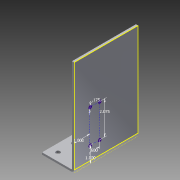
# Autodesk Inventor part: Pneumatic Mount Bracket
Saved by Autodesk Inventor 2013 (Build 170138000, 138)
## iProperties
Created: 2013-02-09
Part Number: Pneumatic Mount Bracket
Material: Aluminum 6061
Document SubType Name: Sheet Metal
Designer: Moses
Mass: 172.904 g
Surface Area: 422.955 cm^2
Volume: 63.8022 cm^3
Density: 2.71 g/cm^3
Sheet Metal Rule: Default
Author: Moses
Autodesk Inventor part; units mm, degrees
ref_plane "YZ Plane" through (0, 0, 0) normal (1, 0, 0) x (0, 1, 0)
ref_plane "XZ Plane" through (0, 0, 0) normal (0, 1, 0) x (-1, 0, 0)
ref_plane "XY Plane" through (0, 0, 0) normal (0, 0, 1) x (1, 0, 0)
sketch "Sketch1" plane through (0, 0, 0) normal (0, 1, 0) x (-1, 0, 0)
  line L0 (0, 0) -> (25.4, 0)
  line L1 (25.4, 0) -> (25.4, 101.6)
  line L2 (25.4, 101.6) -> (0, 101.6)
  line L3 (0, 101.6) -> (0, 0)
  line L4 (12.7, 101.6) -> (12.7, 0) construction
  circle A0 centre (12.7, 12.7) radius 3.302
  circle A1 centre (12.7, 63.5) radius 3.302
  circle A2 centre (12.7, 88.9) radius 3.302
  line L5 (0, 0) -> (-25.4, 0)
  line L6 (-25.4, 0) -> (-25.4, 101.6)
  line L7 (-25.4, 101.6) -> (0, 101.6)
  dimension "d0" = 101.6
  dimension "d2" = 25.4
  dimension "d3" = 6.604
  dimension "d4" = 25.4
  dimension "d5" = 50.8
  dimension "d6" = 12.7
  dimension "d8" = 25.4
  measures "d0" distance of L0.end L1.end
  measures "d2" distance of L0.start L0.end
  measures "d3" diameter of A2
  measures "d4" distance of A1.centre A2.centre
  measures "d5" distance of A0.centre A1.centre
  measures "d6" distance of L4.end A0.centre
  measures "d8" distance of L0.start L5.end
extrude "Plate1" add sketch "Sketch1" along normal blind 3.175
sketch "Sketch2" plane through (22.225, 0, 0) normal (1, 0, 0) x (0, 1, 0)
  line L0 (0, 101.6) -> (0, 0)
  line L1 (0, 0) -> (152.4, 0)
  line L2 (152.4, 0) -> (152.4, 101.6)
  line L3 (152.4, 101.6) -> (0, 101.6)
  constraints: 6 end point, 1 horizontal, 1 perpendicular, 1 vertical
edge flange "Flange1" height 152.4 angle 90 thickness 3.175 bend radius 1.27 thickness toward (1, 0, 0) relief tear relief width 3.175 relief depth 1.5875 edges at (25.4, 3.175, 50.8) wall of the first edge with corners at (22.225, 0, 101.6) (22.225, 0, 0) (22.225, 152.4, 0) (22.225, 152.4, 101.6)
bend "Bend1"
corner "Corner1"
sketch "Sketch3" plane through (25.4, 152.4, 101.6) normal (1, 0, 0) x (0, 0, -1)
  line L0 (0, -147.955) -> (101.6, -147.955) projected
  line L1 (101.6, 0) -> (101.6, -147.955) projected
  line L2 (0, 0) -> (101.6, 0) projected
  line L3 (0, -147.955) -> (0, 0) projected
  line L4 (25.4, -74.295) -> (40.64, -74.295) construction
  line L5 (40.64, -74.295) -> (40.64, -127) construction
  line L6 (40.64, -127) -> (25.4, -127) construction
  line L7 (25.4, -127) -> (25.4, -74.295) construction
  circle A0 centre (25.4, -74.295) radius 2.2225
  circle A1 centre (40.64, -74.295) radius 2.2225
  circle A2 centre (40.64, -127) radius 2.2225
  circle A3 centre (25.4, -127) radius 2.2225
  line L8 (101.6, -152.4) -> (0, -152.4) construction
  dimension "d19" = 52.705
  dimension "d21" = 15.24
  dimension "d22" = 4.445
  dimension "d23" = 25.4
  dimension "d24" = 25.4
  constraints: 8 end point, 4 centre point, 4 coincident, 3 equal radius, 2 parallel, 1 horizontal, 1 perpendicular
  measures "d19" distance of L4.end L5.end
  measures "d21" distance of L5.end L6.end
  measures "d22" diameter of A0
  measures "d23" distance between parallel lines of L8 L6
  measures "d24" distance between parallel lines of L3 L7
equation "\"d9\" = BendReliefWidth"
equation "\"d10\" = BendReliefDepth"
equation "\"d11\" = MinimumRemnant"
equation "\"d12\" = BendRadius"
equation "\"d16\" = CornerReliefSize"
equation "\"d17\" = GapSize"
equation "\"d18\" = JacobiRadiusSize"
equation "\"BendRadius\" = Thickness"
equation "\"BendReliefWidth\" = Thickness"
equation "\"BendReliefDepth\" = 0.5 * Thickness"
equation "\"CornerReliefSize\" = 4 * Thickness"
equation "\"MinimumRemnant\" = 2 * Thickness"
equation "\"TransitionRadius\" = BendRadius"
equation "\"JacobiRadiusSize\" = Thickness"
equation "\"GapSize\" = Thickness"
equation "\"d7\" = BendRadius"
equation "\"Thickness\" = 3.175"
body "Solid1"
